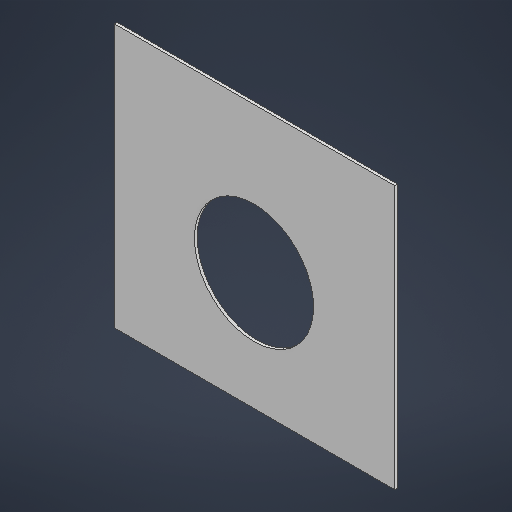
# Autodesk Inventor part: второй верх
Saved by Autodesk Inventor 2026.2 (Build 302298000, 298)
## iProperties
Created: 2025-11-21
Part Number: второй верх
Material: Типовые
Document SubType Name: Modeling
Designer: Phantom
Density: 1 g/cm^3
Appearance: По умолчанию
Author: Phantom
Autodesk Inventor part; units mm, degrees
ref_plane "YZ Plane" through (0, 0, 0) normal (1, 0, 0) x (0, 1, 0)
ref_plane "XZ Plane" through (0, 0, 0) normal (0, 1, 0) x (-1, 0, 0)
ref_plane "XY Plane" through (0, 0, 0) normal (0, 0, 1) x (1, 0, 0)
sketch "Эскиз1" plane through (0, 0, 0) normal (0, 0, 1) x (1, 0, 0)
  line L0 (-202.5, -190) -> (202.5, -190)
  line L1 (202.5, -190) -> (202.5, 190)
  line L2 (202.5, 190) -> (-202.5, 190)
  line L3 (-202.5, 190) -> (-202.5, -190)
  line L4 (-202.5, -190) -> (202.5, 190) construction
  line L5 (202.5, -190) -> (-202.5, 190) construction
  point P0 (0, 0)
  dimension "d0" = 405
  dimension "d1" = 380
  constraints: 12 end point, 2 midpoint, 2 parallel, 1 horizontal, 1 perpendicular
  measures "d0" distance of L2.end L1.end
  measures "d1" distance of L1.end L0.end
extrude "Выдавливание1" add sketch "Эскиз1" along normal blind 4
sketch "Эскиз2" plane through (0, 0, 4) normal (0, 0, 1) x (1, 0, 0)
  line L0 (-202.5, -190) -> (202.5, -190) projected
  line L1 (80, -190) -> (-80, -190)
  circle A0 centre (-0.87, -20.3549) radius 67.5 projected
  point P0 (0, 0)
  point P1 (0, -80)
  constraints: 2 end point, 1 point on line
extrude "Выдавливание2" cut sketch "Эскиз2" against normal blind 10
sketch "Эскиз3" plane through (0, 0, 0) normal (0, 0, -1) x (-1, 0, 0)
  circle A0 centre (0.87, -20.3549) radius 67.5 projected
  circle A1 centre (0.87, -20.3549) radius 80
  point P0 (0, 0)
  dimension "d8" = 160
  constraints: 1 centre point, 1 coincident
  measures "d8" diameter of A1
extrude "Выдавливание3" cut sketch "Эскиз3" against normal blind 10 contours A0 | A1
sketch "Эскиз4" plane through (0, 0, 0) normal (0, 0, -1) x (-1, 0, 0)
  circle A0 centre (-61.1233, -73.4234) radius 2.15 projected
  circle A1 centre (0.87, -20.3549) radius 80 projected
  circle A2 centre (0.87, -20.3549) radius 81.6053
  circle A3 centre (-61.1233, -73.4234) radius 4.5
  circle A4 centre (0.87, -20.3549) radius 86
  point P0 (0, 0)
  dimension "d11" = 9
  dimension "d13" = 172
  constraints: 3 coincident, 2 centre point, 3 other
  measures "d11" diameter of A3
  measures "d13" diameter of A4
extrude "Выдавливание4" cut sketch "Эскиз4" against normal blind 9 contours A0 A1 | A0 A1 A3 | A1 A0 A2 | A0 A2 A3 A1 | A1 A3 A2 A0 | A2 A0 | A0 A2 A3 A4 | A3 A2 A1 | A1 A3 | A3 A4 A2
sketch "Эскиз5" plane through (0, 0, 4) normal (0, 0, 1) x (1, 0, 0)
  line L0 (29.9071, 104.345) -> (29.9071, 34.345) projected
  line L1 (54.63, -143.2364) -> (54.63, -104.4746) projected
  circle A0 centre (-0.87, -20.3549) radius 86 projected
  circle A1 centre (-0.87, -20.3549) radius 150
  line L2 (-79.2827, -52.318) -> (-79.2827, 70.0459) projected
  circle A2 centre (-79.2827, 8.864) radius 61.1819
  circle A3 centre (-0.0936, -20) radius 3.5 projected
  circle A4 centre (-0.0936, -20) radius 150.042
  circle A5 centre (131.7561, -125.6612) radius 19.349
  circle A6 centre (-0.0936, -20) radius 101.8508
  line L3 (131.7561, -125.6612) -> (-0.0936, -20)
  line L4 (131.7561, -125.6612) -> (172.0961, -157.9887)
  line L5 (131.7561, -125.6612) -> (135.6578, -128.7879)
  point P0 (0, 0)
  dimension "d16" = 300
  dimension "d18" = 5
  constraints: 6 end point, 4 centre point, 4 coincident, 1 collinear, 1 midpoint, 1 point on line, 1 tangent, 1 vertical alignment, 2 other
  measures "d16" diameter of A1
  measures "d18" distance of L3.start L5.end
sketch "Эскиз6" plane through (0, 0, 4) normal (0, 0, 1) x (1, 0, 0)
  circle A0 centre (-0.87, -20.3549) radius 86 projected
  circle A1 centre (-0.87, -20.3549) radius 115
  circle A2 centre (-0.87, -20.3549) radius 86 projected
  line L0 (202.5, -190) -> (202.5, 190) projected
  line L1 (202.5, 190) -> (-202.5, 190) projected
  line L2 (-202.5, 190) -> (-202.5, -190) projected
  line L3 (-202.5, -190) -> (202.5, -190) projected
  point P0 (0, 0)
  dimension "d19" = 230
  constraints: 1 centre point, 1 coincident
  measures "d19" diameter of A1
equation "\"d14\" = d11"
